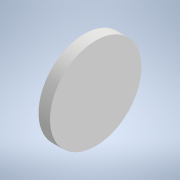
# Autodesk Inventor part: plateForBall
Saved by Autodesk Inventor 2020.2 (Build 242310000, 310)
## iProperties
Created: 2020-01-14
Part Number: plateForBall
Material: Generic
Document SubType Name: Modeling
Designer: steele
Density: 1 g/cm^3
Appearance: Default
Author: steele
Autodesk Inventor part; units mm, degrees
ref_plane "YZ Plane" through (0, 0, 0) normal (1, 0, 0) x (0, 1, 0)
ref_plane "XZ Plane" through (0, 0, 0) normal (0, 1, 0) x (-1, 0, 0)
ref_plane "XY Plane" through (0, 0, 0) normal (0, 0, 1) x (1, 0, 0)
sketch "Sketch1" plane through (0, 0, 0) normal (1, 0, 0) x (0, 1, 0)
  circle A0 centre (0, 0) radius 50.8
  dimension "d0" = 101.6
  constraints: 1 centre point, 1 coincident
  measures "d0" diameter of A0
extrude "Extrusion1" add sketch "Sketch1" along normal mid plane 12.7
sketch "Sketch2" plane through (0, 0, 0) normal (0, 0, 1) x (1, 0, 0)
  arc A0 (22.2941, 50.8) -> (22.2941, -50.8) centre (95.25, 0) ccw
  line L0 (-6.35, 50.8) -> (6.35, 50.8) construction
  line L1 (0, 50.8) -> (0, -50.8) construction
  line L2 (-6.35, 50.8) -> (-6.35, -50.8) construction
  line L3 (6.35, -50.8) -> (6.35, 50.8) projected
  line L4 (0, 0) -> (124.0858, 0) construction
  line L5 (6.35, 50.8) -> (22.2941, 50.8)
  line L6 (6.35, -50.8) -> (22.2941, -50.8)
  point P0 (6.35, 0)
  dimension "d3" = 177.8
  dimension "d4" = 95.25
  dimension "d5" = 0
  constraints: 8 end point, 2 horizontal, 2 point on circle, 1 centre point, 1 midpoint, 1 parallel
  measures "d3" diameter of A0
  measures "d4" distance from line of L1 A0.centre
  measures "d5" distance from line of A0.centre L4
revolve "Revolution1" add sketch "Sketch2" angle 180 about axis through (0, 0, 0) along (1, 0, 0)
sketch "Sketch3" plane through (-6.35, 0, 0) normal (-1, 0, 0) x (0, 0, 1)
  circle A0 centre (0, 0) radius 4.2164
  dimension "d7" = 8.4328
  constraints: 1 centre point, 1 coincident
  measures "d7" diameter of A0
extrude "Extrusion2" cut sketch "Sketch3" against normal blind 12.7
body "Solid1"
